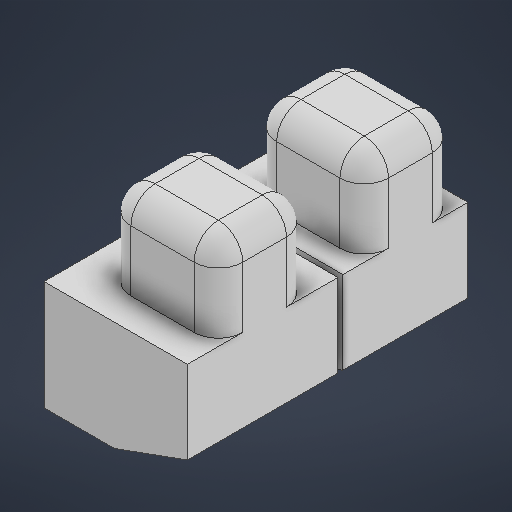
# Autodesk Inventor part: botones
Saved by Autodesk Inventor 2027 (Build 310192000, 192)
## iProperties
Created: 2026-06-02
Part Number: botones
Material: Generic
Document SubType Name: Modeling
Designer: Administrador
Density: 1 g/cm^3
Appearance: Default
Author: Administrador
Autodesk Inventor part; units mm, degrees
ref_plane "YZ Plane" through (0, 0, 0) normal (1, 0, 0) x (0, 1, 0)
ref_plane "XZ Plane" through (0, 0, 0) normal (0, 1, 0) x (-1, 0, 0)
ref_plane "XY Plane" through (0, 0, 0) normal (0, 0, 1) x (1, 0, 0)
sketch "Sketch1" plane through (0, 0, 0) normal (0, 1, 0) x (-1, 0, 0)
  line L0 (2.0875, 6.0669) -> (-2.5125, 6.0669)
  line L1 (-2.5125, 6.0669) -> (-2.5125, 2.2669)
  line L2 (-2.5125, 2.2669) -> (2.0875, 2.2669)
  line L3 (2.0875, 2.2669) -> (2.0875, 6.0669)
  line L4 (2.0875, 6.0669) -> (-2.5125, 2.2669) construction
  line L5 (-2.5125, 6.0669) -> (2.0875, 2.2669) construction
  line L6 (-2.5125, -3.7331) -> (2.0875, -3.7331)
  line L7 (2.0875, -3.7331) -> (2.0875, 0.0669)
  line L8 (2.0875, 0.0669) -> (-2.5125, 0.0669)
  line L9 (-2.5125, 0.0669) -> (-2.5125, -3.7331)
  line L10 (-2.5125, -3.7331) -> (2.0875, 0.0669) construction
  line L11 (2.0875, -3.7331) -> (-2.5125, 0.0669) construction
  point P0 (0, 0)
  point P1 (2.8581, 5.0437)
  point P2 (-0.2125, 4.1669)
  point P3 (-0.2125, -1.8331)
  point P4 (-0.2125, 0.0669)
  point P5 (-0.2125, 2.2669)
  dimension "d0" = 3.8
  dimension "d1" = 3.8
  dimension "d2" = 4.6
  dimension "d3" = 4.6
  dimension "d4" = 6
  constraints: 24 end point, 6 midpoint, 4 parallel, 2 horizontal, 2 perpendicular
  measures "d0" distance of L2.end L0.start
  measures "d1" distance of L6.end L7.end
  measures "d2" distance of L6.start L6.end
  measures "d3" distance of L0.start L0.end
  measures "d4" distance of point (-0.213, -1.833) point (-0.213, 4.167)
extrude "Extrusion1" add sketch "Sketch1" against normal blind 8
fillet "Fillet1" radius 1 5 edges at (-2.0875, -4, 6.0669) (2.5125, -4, 6.0669) (2.5125, -4, 2.2669) (2.5125, -4, 0.0669) (2.5125, -4, -3.7331)
fillet "Fillet2" radius 1 3 edges at (-2.0875, -4, 2.2669) (-2.0875, -4, -3.7331) (-2.0875, -4, 0.0669)
fillet "Fillet3" radius 1 16 edges at (-1.7946, 0, 2.5598) (-2.0875, 0, 4.1669) (-1.7946, 0, 5.774) (0.2125, 0, 6.0669) (2.2196, 0, 5.774) (2.5125, 0, 4.1669) (2.2196, 0, 2.5598) (0.2125, 0, 2.2669) (-1.7946, 0, -3.4402) (-2.0875, 0, -1.8331) (-1.7946, 0, -0.226) (0.2125, 0, 0.0669) (2.2196, 0, -0.226) (2.5125, 0, -1.8331) (2.2196, 0, -3.4402) (0.2125, 0, -3.7331)
sketch "Sketch2" plane through (0, -8, 0) normal (0, -1, 0) x (1, 0, 0)
  point P0 (0, 0)
sketch "Sketch3" plane through (0, -8, 0) normal (0, -1, 0) x (1, 0, 0)
  line L0 (-3.387, 0.9432) -> (2.5125, 0.9432)
  line L1 (2.5125, 0.9432) -> (2.5125, -4.2017)
  line L2 (2.5125, -4.2017) -> (-3.387, -4.2017)
  line L3 (-3.387, -4.2017) -> (-3.387, 0.9432)
  line L4 (-3.387, 1.149) -> (2.5125, 1.149)
  line L5 (2.5125, 1.149) -> (2.5125, 7.3401)
  line L6 (2.5125, 7.3401) -> (-3.387, 7.3401)
  line L7 (-3.387, 7.3401) -> (-3.387, 1.149)
  line L8 (2.5125, -0.9331) -> (2.5125, -2.7331) projected
  line L9 (2.5125, 5.0669) -> (2.5125, 3.2669) projected
  point P0 (0, 0)
  point P1 (2.5125, -1.8331)
  point P2 (2.5125, 4.1669)
  point P3 (2.5125, 4.2446)
  dimension "d16" = 5.8995
  dimension "d17" = 5.1449
  dimension "d18" = 6.191
  dimension "d19" = 0
  dimension "d20" = 0
  constraints: 16 end point, 4 parallel, 3 midpoint, 2 horizontal, 2 perpendicular
  measures "d16" distance of L1.end L2.end
  measures "d17" distance of L0.end L1.end
  measures "d18" distance of L4.end L5.end
  measures "d19" distance from line of point (2.513, -1.833) L1
  measures "d20" horizontal distance of point (2.513, 4.167) point (2.513, 4.245)
extrude "Extrusion2" add sketch "Sketch3" against normal blind 4.5
chamfer "Chamfer1" distance 3 angle 20 1 edges at (2.5125, -8, 4.2446) measured on face at (0.546, -8, 3.2127)
chamfer "Chamfer2" distance 3 angle 20 1 edges at (2.5125, -8, -1.6292) measured on face at (-1.4205, -8, -0.7717)
body "Solid1"
